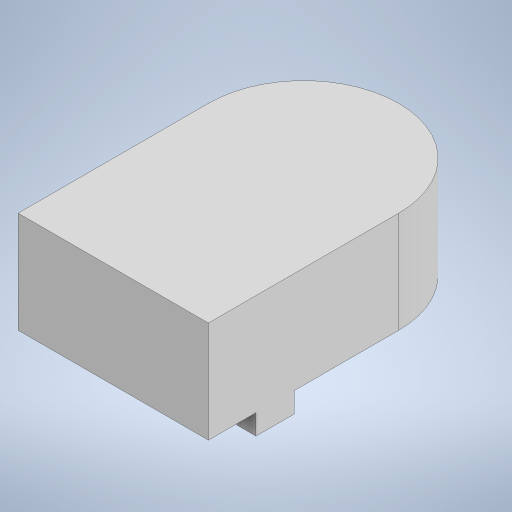
# Autodesk Inventor part: ANDGATE
Saved by Autodesk Inventor 2023 (Build 270158000, 158)
## iProperties
Created: 2024-01-22
Part Number: ANDGATE
Material: Generic
Document SubType Name: Modeling
Designer: Jetsan
Density: 1 g/cm^3
Appearance: Default
Author: Jetsan
Autodesk Inventor part; units mm, degrees
ref_plane "YZ Plane" through (0, 0, 0) normal (1, 0, 0) x (0, 1, 0)
ref_plane "XZ Plane" through (0, 0, 0) normal (0, 1, 0) x (-1, 0, 0)
ref_plane "XY Plane" through (0, 0, 0) normal (0, 0, 1) x (1, 0, 0)
sketch "Sketch1" plane through (0, 0, 0) normal (0, 1, 0) x (-1, 0, 0)
  line L0 (-7.5, 7.5) -> (7.5, 7.5)
  line L1 (7.5, 7.5) -> (7.5, -7.5)
  line L2 (7.5, -7.5) -> (-7.5, -7.5)
  line L3 (-7.5, -7.5) -> (-7.5, 7.5)
  line L4 (-7.5, 7.5) -> (7.5, -7.5) construction
  line L5 (7.5, 7.5) -> (-7.5, -7.5) construction
  circle A0 centre (0, -7.5) radius 7.5 construction
  arc A1 (-7.5, -7.5) -> (7.5, -7.5) centre (0, -7.5) ccw
  point P0 (0, 0)
  dimension "d0" = 15
  dimension "d1" = 15
  constraints: 12 end point, 3 midpoint, 2 parallel, 2 point on circle, 1 centre point, 1 coincident, 1 horizontal, 1 horizontal alignment, 1 perpendicular, 2 other
  measures "d0" distance of L0.end L1.end
  measures "d1" distance of L0.start L0.end
extrude "Extrusion1" add sketch "Sketch1" along normal blind 8
sketch "Sketch2" plane through (0, 0, 0) normal (0, -1, 0) x (1, 0, 0)
  line L0 (7.5, 11.25) -> (-7.5, 11.25)
  line L1 (-7.5, 11.25) -> (-7.5, -18.75)
  line L2 (-7.5, -18.75) -> (7.5, -18.75)
  line L3 (7.5, -18.75) -> (7.5, 11.25)
  line L4 (7.5, 11.25) -> (-7.5, -18.75) construction
  line L5 (-7.5, 11.25) -> (7.5, -18.75) construction
  line L6 (-7.5, 7.5) -> (7.5, 7.5) projected
  line L7 (7, 10.75) -> (-7, 10.75) construction
  line L8 (-7, 10.75) -> (-7, -18.25) construction
  line L9 (-7, -18.25) -> (7, -18.25) construction
  line L10 (7, -18.25) -> (7, 10.75) construction
  line L11 (7, 10.75) -> (-7, -18.25) construction
  line L12 (-7, 10.75) -> (7, -18.25) construction
  point P0 (0, 0)
  point P1 (0, -3.75)
  dimension "d4" = 15
  dimension "d5" = 30
  dimension "d6" = 3.75
  dimension "d18" = 0.5
  dimension "d19" = 0.5
  constraints: 24 end point, 4 midpoint, 4 parallel, 2 horizontal, 2 perpendicular
  measures "d4" distance of L2.end L1.end
  measures "d5" distance of L1.end L0.end
  measures "d6" distance between parallel lines of L0 L6
  measures "d18" distance between parallel lines of L2 L9
  measures "d19" distance between parallel lines of L3 L10
sketch "Sketch4" plane through (0, 0, 0) normal (0, -1, 0) x (1, 0, 0)
  line L0 (-7.5, -7.5) -> (-7.5, 7.5) projected
  line L1 (-7.5, 3.75) -> (-6, 3.75)
  line L2 (-6, 3.75) -> (-6, 0.75)
  line L3 (-6, 0.75) -> (-7.5, 0.75)
  line L4 (-7.5, 0.75) -> (-7.5, 3.75)
  line L5 (7.5, 7.5) -> (7.5, -7.5) projected
  line L6 (7.5, 0.75) -> (6, 0.75)
  line L7 (6, 0.75) -> (6, 3.75)
  line L8 (6, 3.75) -> (7.5, 3.75)
  line L9 (7.5, 3.75) -> (7.5, 0.75)
  line L10 (-7.5, -18.75) -> (7.5, -18.75) construction
  line L11 (7.5, -18.75) -> (7.5, 11.25) construction
  line L12 (7.5, 11.25) -> (-7.5, 11.25) construction
  line L13 (-7.5, 11.25) -> (-7.5, -18.75) construction
  line L14 (-7.5, -18.75) -> (7.5, 11.25) construction
  line L15 (7.5, -18.75) -> (-7.5, 11.25) construction
  line L16 (-7.5, 7.5) -> (7.5, 7.5) construction
  arc A0 (-7.5, -7.5) -> (7.5, -7.5) centre (0, -7.5) ccw construction
  point P0 (0, 0)
  point P1 (0, -3.75)
  point P2 (0, -15)
  point P3 (-6.75, 3.75)
  point P4 (7.5, 3.75)
  dimension "d20" = 1.5
  dimension "d21" = 3
  dimension "d22" = 1.5
  dimension "d23" = 3
  dimension "d24" = 15
  dimension "d25" = 30
  dimension "d26" = 3.75
  dimension "d27" = 3.75
  dimension "d28" = 7.5
  constraints: 28 end point, 6 parallel, 3 horizontal, 3 midpoint, 3 perpendicular, 3 point on line, 1 point on circle
  measures "d20" distance of L2.end L3.end
  measures "d21" distance of L1.end L2.end
  measures "d22" distance of L7.end L8.end
  measures "d23" distance of L6.end L7.end
  measures "d24" distance of L12.end L11.end
  measures "d25" distance of L11.end L10.end
  measures "d26" distance between parallel lines of L16 L12
  measures "d27" distance from line of L10 point (0, -15)
  measures "d28" distance from line of L12 point (-6.75, 3.75)
extrude "Extrusion3" add sketch "Sketch4" along normal blind 1.6
sketch "Sketch6" plane through (0, 0, 0) normal (0, -1, 0) x (1, 0, 0)
  line L0 (7.5, 11.25) -> (-7.5, 11.25)
  line L1 (-7.5, 11.25) -> (-7.5, -18.75)
  line L2 (-7.5, -18.75) -> (7.5, -18.75)
  line L3 (7.5, -18.75) -> (7.5, 11.25)
  line L4 (7.5, 11.25) -> (-7.5, -18.75) construction
  line L5 (-7.5, 11.25) -> (7.5, -18.75) construction
  line L6 (7, 10.75) -> (-7, 10.75) construction
  line L7 (-7, 10.75) -> (-7, -18.25) construction
  line L8 (-7, -18.25) -> (7, -18.25) construction
  line L9 (7, -18.25) -> (7, 10.75) construction
  line L10 (7, 10.75) -> (-7, -18.25) construction
  line L11 (-7, 10.75) -> (7, -18.25) construction
  circle A0 centre (0, -3.75) radius 1.25
  circle A1 centre (0, -3.75) radius 1.75
  line L12 (-7, 7) -> (7, 7)
  line L13 (7, 7) -> (7, -7.5)
  line L14 (7, -7.5) -> (-7, -7.5)
  line L15 (-7, -7.5) -> (-7, 7)
  line L16 (-7.5, 7.5) -> (7.5, 7.5) projected
  arc A2 (-7.5, -7.5) -> (7.5, -7.5) centre (0, -7.5) ccw projected
  circle A3 centre (0, -7.5) radius 7
  point P0 (0, 0)
  point P1 (-7.5, -3.75)
  point P2 (7, -7.5)
  dimension "d31" = 15
  dimension "d32" = 30
  dimension "d34" = 0.5
  dimension "d35" = 0.5
  dimension "d36" = 2.5
  dimension "d37" = 0.5
  dimension "d38" = 0.5
  dimension "d39" = 0.5
  dimension "d40" = 0.5
  dimension "d41" = 0.5
  constraints: 32 end point, 6 parallel, 5 midpoint, 3 coincident, 3 horizontal, 3 perpendicular, 2 centre point, 3 other
  measures "d31" distance of L2.end L1.end
  measures "d32" distance of L1.end L0.end
  measures "d34" distance between parallel lines of L2 L8
  measures "d35" distance between parallel lines of L3 L9
  measures "d36" diameter of A0
  measures "d37" radial gap between concentric circles of A0 A1
  measures "d38" distance between parallel lines of L16 L12
  measures "d39" distance from line of point (-7.5, -3.75) L15
  measures "d40" distance between parallel lines of L3 L13
extrude "Extrusion4" cut sketch "Sketch6" against normal blind 5 contours A0 | L12 L13 A3 L15 | A3 L14 | L14 A3
sketch "Sketch7" plane through (0, 5, -3.75) normal (0, -1, 0) x (1, 0, 0)
  circle A0 centre (0, 0) radius 1.25
  point P0 (0, 3.75)
  constraints: 1 centre point
body "Solid1"
